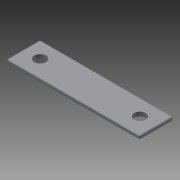
# Autodesk Inventor part: 4 hole long poly
Saved by Autodesk Inventor 2014 SP1 (Build 180222100, 222)
## iProperties
Created: 2014-02-27
Part Number: 4 hole long poly
Material: Generic
Document SubType Name: Modeling
Designer: Ryan
Density: 1 g/cm^3
Appearance: Default
Author: Ryan
Autodesk Inventor part; units mm, degrees
ref_plane "YZ Plane" through (0, 0, 0) normal (1, 0, 0) x (0, 1, 0)
ref_plane "XZ Plane" through (0, 0, 0) normal (0, 1, 0) x (-1, 0, 0)
ref_plane "XY Plane" through (0, 0, 0) normal (0, 0, 1) x (1, 0, 0)
sketch "Sketch1" plane through (0, 0, 0) normal (0, 1, 0) x (-1, 0, 0)
  line L0 (-27.8977, 8.1703) -> (22.9023, 8.1703)
  line L1 (22.9023, 8.1703) -> (22.9023, -4.5297)
  line L2 (22.9023, -4.5297) -> (-27.8977, -4.5297)
  line L3 (-27.8977, -4.5297) -> (-27.8977, 8.1703)
  point P0 (0, 0)
  dimension "d0" = 50.8
  dimension "d1" = 12.7
  constraints: 8 end point, 2 parallel, 1 horizontal, 1 perpendicular
  measures "d0" distance of L1.end L2.end
  measures "d1" distance of L0.end L1.end
extrude "Extrusion1" add sketch "Sketch1" along normal blind 1.5875
sketch "Sketch2" plane through (0, 1.5875, 0) normal (0, 1, 0) x (1, 0, 0)
  line L0 (27.8977, -8.1703) -> (27.8977, 4.5297) projected
  line L1 (27.8977, 4.5297) -> (-22.9023, 4.5297) projected
  line L2 (-22.9023, 4.5297) -> (-22.9023, -8.1703) projected
  circle A0 centre (-16.5523, -1.8203) radius 2.2225
  circle A1 centre (21.5477, -1.8203) radius 2.2225
  point P0 (0, 0)
  dimension "d4" = 4.445
  dimension "d5" = 6.35
  dimension "d6" = 4.445
  dimension "d7" = 6.35
  dimension "d8" = 6.35
  dimension "d9" = 6.35
  constraints: 2 centre point
  measures "d4" diameter of A0
  measures "d5" distance from line of L2 A0.centre
  measures "d6" diameter of A1
  measures "d7" distance from line of L0 A1.centre
  measures "d8" distance from line of A1.centre L1
  measures "d9" distance from line of L1 A0.centre
extrude "Extrusion2" cut sketch "Sketch2" against normal blind 1.5875
fillet "Fillet1" radius 0.508 12 edges at (2.4977, 1.5875, 8.1703) (-22.9023, 0, 1.8203) (-22.9023, 0.7937, 8.1703) (-22.9023, 1.5875, 1.8203) (-22.9023, 0.7937, -4.5297) (2.4977, 0, -4.5297) (2.4977, 1.5875, -4.5297) (27.8977, 0.7937, -4.5297) (27.8977, 0, 1.8203) (27.8977, 1.5875, 1.8203) (27.8977, 0.7937, 8.1703) (2.4977, 0, 8.1703)
body "Solid1"
